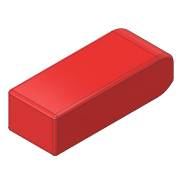
# Autodesk Inventor part: KYPOM_K6_4S1500MAH
Saved by Autodesk Inventor 2019.4 (Build 234330000, 330)
## iProperties
Created: 2019-11-23
Part Number: KYPOM_K6_4S1500MAH
Material: 一般
Document SubType Name: Modeling
Designer: y6tada
Density: 1 g/cm^3
Appearance: 淡い赤
Author: y6tada
Autodesk Inventor part; units mm, degrees
ref_plane "YZ Plane" through (0, 0, 0) normal (1, 0, 0) x (0, 1, 0)
ref_plane "XZ Plane" through (0, 0, 0) normal (0, 1, 0) x (-1, 0, 0)
ref_plane "XY Plane" through (0, 0, 0) normal (0, 0, 1) x (1, 0, 0)
sketch "スケッチ1" plane through (0, 0, 0) normal (1, 0, 0) x (0, 0, -1)
  line L0 (-42.5, 12.75) -> (32.0388, 12.75)
  line L1 (42.5, 12.75) -> (42.5, 8.5) construction
  line L2 (42.5, -12.75) -> (32.0388, -12.75) construction
  line L3 (-42.5, -12.75) -> (-42.5, 12.75)
  line L4 (0, 0) -> (44.8735, 0) construction
  line L5 (0, 0) -> (0, 24.3988) construction
  arc A0 (42.5, 8.5) -> (32.0388, 12.75) centre (32.0388, -2.25) ccw
  arc A1 (32.0388, -12.75) -> (42.5, -8.5) centre (32.0388, 2.25) ccw
  line L6 (32.0388, 12.75) -> (42.5, 12.75) construction
  line L7 (42.5, 8.5) -> (42.5, -8.5)
  line L8 (42.5, -8.5) -> (42.5, -12.75) construction
  line L9 (32.0388, -12.75) -> (-42.5, -12.75)
  dimension "d0" = 85
  dimension "d1" = 25.5
  dimension "d4" = 15
  dimension "d5" = 17
  constraints: 20 end point, 7 parallel, 6 perpendicular, 4 point on circle, 4 tangent, 3 horizontal, 2 centre point, 1 equal radius, 1 point on line, 1 symmetric about line, 1 vertical, 2 other
  measures "d0" distance of L0.start L1.start
  measures "d1" distance of L1.start L2.start
  measures "d4" radius of A0
  measures "d5" distance of L7.end L1.end
extrude "押し出し1" add sketch "スケッチ1" along normal mid plane 35
fillet "フィレット1" radius 2 12 edges at (0, 12.75, 42.5) (17.5, 0, 42.5) (17.5, 11.6469, -37.6846) (17.5, 12.75, 5.2306) (-17.5, 0, 42.5) (0, -12.75, 42.5) (17.5, -11.6469, -37.6846) (17.5, -12.75, 5.2306) (-17.5, -11.6469, -37.6846) (-17.5, -12.75, 5.2306) (-17.5, 11.6469, -37.6846) (-17.5, 12.75, 5.2306)
